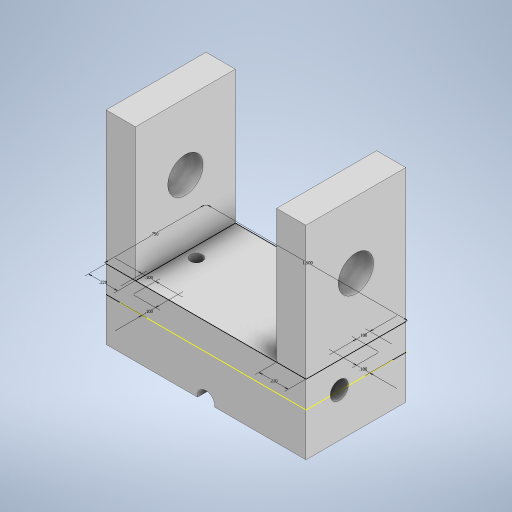
# Autodesk Inventor part: HomemadeSensorHousing 8020
Saved by Autodesk Inventor 2024.1 (Build 281209000, 209)
## iProperties
Created: 2022-02-14
Part Number: HomemadeSensorHousing 8020
Material: Generic
Document SubType Name: Modeling
Designer: Beaucage
Density: 1 g/cm^3
Appearance: Default
Author: Beaucage
Autodesk Inventor part; units mm, degrees
ref_plane "YZ Plane" through (0, 0, 0) normal (1, 0, 0) x (0, 1, 0)
ref_plane "XZ Plane" through (0, 0, 0) normal (0, 1, 0) x (-1, 0, 0)
ref_plane "XY Plane" through (0, 0, 0) normal (0, 0, 1) x (1, 0, 0)
sketch "Sketch1" plane through (0, 0, 0) normal (0, 1, 0) x (-1, 0, 0)
  line L0 (0, 0) -> (38.1, 0)
  line L1 (38.1, 0) -> (38.1, -19.05)
  line L2 (38.1, -19.05) -> (0, -19.05)
  line L3 (0, -19.05) -> (0, 0)
  line L4 (38.1, -19.05) -> (32.512, -19.05)
  line L5 (32.512, -19.05) -> (32.512, 0)
  line L6 (32.512, 0) -> (38.1, 0)
  line L7 (38.1, 0) -> (38.1, -19.05)
  line L8 (0, -19.05) -> (5.588, -19.05)
  line L9 (5.588, -19.05) -> (5.588, 0)
  line L10 (5.588, 0) -> (0, 0)
  line L11 (0, 0) -> (0, -19.05)
  point P0 (5.588, -19.05)
  dimension "d0" = 38.1
  dimension "d1" = 19.05
  dimension "d2" = 5.588
  dimension "d3" = 5.588
  constraints: 24 end point, 6 parallel, 3 horizontal, 3 perpendicular, 2 point on line
  measures "d0" distance of L1.end L2.end
  measures "d1" distance of L0.end L1.end
  measures "d2" distance of L5.end L6.end
  measures "d3" distance of L10.end L9.end
extrude "Extrusion1" add sketch "Sketch1" along normal blind 25.4 contours L0 L9 L2 L3 | L0 L1 L2 L5
extrude "Extrusion2" add sketch "Sketch1" against normal blind 5.08
sketch "Sketch2" plane through (0, 25.4, 0) normal (1, 0, 0) x (0, 0, -1)
  line L0 (19.05, 0) -> (0, 0) projected
  line L1 (9.525, 0) -> (9.525, -12.7)
  point P0 (0, -25.4)
  dimension "d8" = 12.7
  constraints: 2 end point, 1 midpoint, 1 vertical
  measures "d8" distance of L1.start L1.end
hole "Hole1" at (0, 12.7, -9.525) direction (-1, 0, 0) diameter 6.7564 end through all start extended yes clearance for "Socket Head Cap Screw" size "1/4" standard "Ansi Unified Screw Threads"
sketch "Sketch3" plane through (0, -5.08, 0) normal (0, -1, 0) x (1, 0, 0)
  line L0 (0, 0) -> (-38.1, 0) projected
  line L1 (-38.1, 0) -> (-35.56, 0)
  line L2 (-35.56, 0) -> (-35.56, -2.54)
  line L3 (-35.56, -2.54) -> (-38.1, -2.54)
  line L4 (-38.1, -2.54) -> (-38.1, 0)
  line L5 (0, -19.05) -> (-2.54, -19.05)
  line L6 (-2.54, -19.05) -> (-2.54, -16.51)
  line L7 (-2.54, -16.51) -> (0, -16.51)
  line L8 (0, -16.51) -> (0, -19.05)
  line L9 (-35.56, -2.54) -> (-2.54, -2.54)
  line L10 (-2.54, -2.54) -> (-2.54, -16.51)
  line L11 (-2.54, -16.51) -> (-35.56, -16.51)
  line L12 (-35.56, -16.51) -> (-35.56, -2.54)
  line L13 (-38.1, 0) -> (-38.1, -19.05) projected
  line L14 (0, -19.05) -> (0, 0) projected
  line L15 (-38.1, -19.05) -> (0, -19.05) projected
  dimension "d16" = 2.54
  dimension "d17" = 2.54
  dimension "d18" = 2.54
  dimension "d19" = 2.54
  constraints: 24 end point, 6 parallel, 3 horizontal, 3 perpendicular
  measures "d16" distance of L2.end L3.end
  measures "d17" distance of L1.end L2.end
  measures "d18" distance of L6.end L7.end
  measures "d19" distance of L5.end L6.end
extrude "Extrusion3" cut sketch "Sketch3" against normal blind 2.54 contours L9 L10 L11 L12
extrude "Extrusion4" add sketch "Sketch3" along normal blind 8.255 contours L14 L7 L10 L9 L2 L0 | L2 L3 L4 L0 | L8 L5 L6 L7 | L12 L11 L6 L15 L13 L3
sketch "Sketch4" plane through (0, 25.4, 0) normal (1, 0, 0) x (0, 0, -1)
  line L0 (19.05, -38.735) -> (19.05, 0) projected
  line L1 (19.05, -30.3802) -> (6.35, -30.3802)
  line L2 (19.05, -30.3802) -> (31.75, -30.3802) construction
  point P0 (0, -25.4)
  dimension "d24" = 12.7
  dimension "d25" = 180
  constraints: 4 end point, 1 collinear, 1 horizontal, 1 perpendicular, 1 point on line
  measures "d24" distance of L1.start L1.end
  measures "d25" angle of L1 L2
hole "Hole2" at (0, -4.9802, -6.35) direction (-1, 0, 0) diameter 3.4544 depth 2.54
sketch "Sketch5" plane through (0, -2.54, 0) normal (0, -1, 0) x (1, 0, 0)
  line L0 (-2.54, -16.51) -> (-35.56, -16.51) projected
  line L1 (-19.05, -16.51) -> (-19.05, -2.54)
  line L2 (-35.56, -2.54) -> (-2.54, -2.54) projected
  line L3 (-35.56, -2.54) -> (-2.54, -2.54) projected
  line L4 (-19.05, -16.51) -> (-19.05, -9.525)
  line L5 (-4.2545, -5.715) -> (-33.8455, -5.715)
  line L6 (-33.8455, -5.715) -> (-33.8455, -13.335)
  line L7 (-33.8455, -13.335) -> (-4.2545, -13.335)
  line L8 (-4.2545, -13.335) -> (-4.2545, -5.715)
  line L9 (-4.2545, -5.715) -> (-33.8455, -13.335) construction
  line L10 (-33.8455, -5.715) -> (-4.2545, -13.335) construction
  line L11 (-19.05, -9.525) -> (-30.4165, -9.525)
  line L12 (-30.4165, -9.525) -> (-7.6835, -9.525)
  point P0 (0, 0)
  dimension "d33" = 6.985
  dimension "d34" = 29.591
  dimension "d35" = 7.62
  dimension "d36" = 11.3665
  dimension "d37" = 22.733
  constraints: 20 end point, 5 midpoint, 2 horizontal, 2 parallel, 1 perpendicular, 1 point on line
  measures "d33" distance of L1.start L4.end
  measures "d34" distance of L7.end L6.end
  measures "d35" distance of L6.end L5.end
  measures "d36" distance of L4.end L11.end
  measures "d37" distance of L11.end L12.end
hole "Hole3" at (-7.6835, -2.54, -9.525) at (-30.4165, -2.54, -9.525) direction (0, 1, 0) diameter 2.2606 end through all
sketch "Sketch6" plane through (-35.56, -2.54, -16.51) normal (0, 0, 1) x (1, 0, 0)
  line L0 (33.02, 0) -> (0, 0) projected
  line L1 (16.51, 0) -> (16.51, -10.541)
  point P0 (35.56, 2.54)
  dimension "d45" = 10.541
  constraints: 2 end point, 1 midpoint, 1 vertical
  measures "d45" distance of L1.start L1.end
hole "Hole4" at (-19.05, -13.081, -16.51) direction (0, 0, 1) diameter 3.302 end through all both
body "Solid1"
